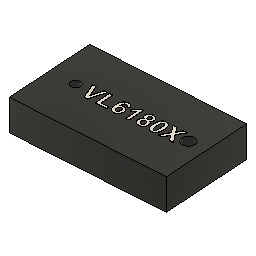
VL6180X Breakout Board v4 (Autodesk Fusion 360 archive; units mm, degrees)
design "VL6180X"
Autodesk Fusion 360 part; units mm, degrees
sketch "Skizze1" plane through (0, 0, 0) normal (0, 1, 0) x (1, 0, 0)
  line L0 (1.4, 2.4) -> (-1.4, 2.4)
  line L1 (-1.4, 2.4) -> (-1.4, -2.4)
  line L2 (-1.4, -2.4) -> (1.4, -2.4)
  line L3 (1.4, -2.4) -> (1.4, 2.4)
  line L4 (1.4, 2.4) -> (-1.4, -2.4) construction
  line L5 (-1.4, 2.4) -> (1.4, -2.4) construction
  line L6 (0, -2.4) -> (0, -1.85) construction
  line L7 (0, 2.4) -> (0, 1.6) construction
  line L8 (-0.1772, 1.2858) -> (-0.1772, -0.3972) construction
  line L9 (-0.1772, -0.3972) -> (0.2288, -0.3972) construction
  line L10 (0.2288, -0.3972) -> (0.2288, 1.2858) construction
  line L11 (0.2288, 1.2858) -> (-0.1772, 1.2858) construction
  circle A0 centre (0, -1.85) radius 0.2
  circle A1 centre (0, 1.6) radius 0.15
  dimension "d1" = 2.8
  dimension "d2" = 4.8
  dimension "d3" = 0.55
  dimension "d4" = 0.8
  dimension "d5" = 0.5
  dimension "d6" = 0.4
  dimension "d7" = 0.3
  text T0 "VL6180X" font "Arial" height 0.5 bold align left top in box 1.683 x 0.406 at (-0.1772, 1.2858) x (0, -1) y (1, 0) spacing 1 kerned
  constraint horizontal L0
  constraint perpendicular L0 L1
  constraint parallel L0 L2
  constraint parallel L1 L3
  constraint coincident L4 origin
  constraint coincident L5 origin
  constraint midpoint L2 L6.start
  constraint perpendicular L2 L6
  constraint midpoint L0 L7.start
  constraint perpendicular L0 L7
  constraint coincident L6.end A0.centre
  constraint coincident L7.end A1.centre
  measures "d1" distance of L1.end L2.end
  measures "d2" distance of L0.end L1.end
  measures "d3" distance of L6.start L6.end
  measures "d4" distance of L7.start L7.end
  measures "d6" diameter of A0
  measures "d7" diameter of A1
extrude "Extrusion1" add sketch "Skizze1" against normal blind 1 contours L0 L1 L2 L3 | A0 | A1 makes body 1
extrude "Extrusion2" cut sketch "Skizze1" against normal blind 0.5 contours A0 | A1 bodies 1
extrude "Extrusion3" add sketch "Skizze1" along normal blind 0.01 separate body text T0 makes body 2 at (-0.0778, 0, -0.7324) makes body 3 at (-0.1854, 0, 1.5283) makes body 4 at (-0.0031, 0, 0.6179) makes body 5 at (-0.0601, 0, 1.0921) makes body 6 at (0.0166, 0, 0.2385) makes body 7 at (-0.0251, 0, -0.2918) makes body 8 at (-0.0612, 0, -1.1476)
